Autodesk Fusion 360 part; units mm, degrees
(part 3 of 3)
  line L801 (-42.271, 19.322) -> (-42.57, 20.092)
  line L802 (-42.57, 20.092) -> (-42.917, 21.434)
  line L803 (-42.917, 21.434) -> (-43.042, 22.229)
  line L804 (-43.042, 22.229) -> (-43.116, 23.149)
  line L805 (-43.116, 23.149) -> (-43.116, 28.119)
  line L806 (-43.116, 28.119) -> (-42.942, 28.168)
  line L807 (-42.942, 28.168) -> (-42.843, 28.342)
  line L808 (-42.843, 28.342) -> (-42.843, 34.257)
  line L809 (-42.843, 34.257) -> (-42.967, 34.406)
  line L810 (-42.967, 34.406) -> (-43.887, 34.406)
  line L811 (-43.887, 34.406) -> (-44.011, 34.282)
  line L812 (-44.011, 34.282) -> (-44.011, 28.268)
  line L813 (-44.011, 28.268) -> (-43.936, 28.168)
  line L814 (-43.936, 28.168) -> (-43.837, 28.119)
  line L815 (-43.837, 28.119) -> (-43.837, 23.323)
  line L816 (-43.837, 23.323) -> (-43.762, 22.279)
  line L817 (-43.762, 22.279) -> (-43.564, 21.061)
  line L818 (-43.564, 21.061) -> (-43.315, 20.092)
  line L819 (-43.315, 20.092) -> (-42.942, 19.073)
  line L820 (-42.942, 19.073) -> (-42.57, 18.303)
  line L821 (-42.57, 18.303) -> (-42.172, 17.632)
  line L822 (-42.172, 17.632) -> (-41.799, 17.11)
  line L823 (-41.799, 17.11) -> (-41.153, 16.389)
  line L824 (-41.153, 16.389) -> (-40.383, 15.743)
  line L825 (-40.383, 15.743) -> (-39.712, 15.321)
  line L826 (-39.712, 15.321) -> (-39.687, 15.246)
  line L827 (-39.687, 15.246) -> (-39.761, 15.196)
  line L828 (-39.761, 15.196) -> (-40.532, 15.221)
  line L829 (-40.532, 15.221) -> (-41.079, 15.296)
  line L830 (-41.079, 15.296) -> (-41.6, 15.42)
  line L831 (-41.6, 15.42) -> (-42.545, 15.793)
  line L832 (-42.545, 15.793) -> (-43.191, 16.166)
  line L833 (-43.191, 16.166) -> (-43.837, 16.663)
  line L834 (-43.837, 16.663) -> (-44.409, 17.234)
  line L835 (-44.409, 17.234) -> (-44.756, 17.657)
  line L836 (-44.756, 17.657) -> (-45.353, 18.576)
  line L837 (-45.353, 18.576) -> (-45.8, 19.496)
  line L838 (-45.8, 19.496) -> (-46.123, 20.365)
  line L839 (-46.123, 20.365) -> (-46.347, 21.161)
  line L840 (-46.347, 21.161) -> (-46.496, 21.906)
  line L841 (-46.496, 21.906) -> (-46.62, 22.95)
  line L842 (-46.62, 22.95) -> (-46.645, 26.205)
  line L843 (-46.645, 26.205) -> (-46.546, 26.28)
  line L844 (-46.546, 26.28) -> (-46.496, 26.379)
  line L845 (-46.496, 26.379) -> (-46.496, 31.747)
  line L846 (-46.496, 31.747) -> (-46.67, 31.871)
  line L847 (-46.67, 31.871) -> (-47.515, 31.846)
  line L848 (-47.515, 31.846) -> (-47.614, 31.722)
  line L849 (-47.614, 31.722) -> (-47.614, 26.379)
  line L850 (-47.614, 26.379) -> (-47.54, 26.255)
  line L851 (-47.54, 26.255) -> (-47.416, 26.23)
  line L852 (-47.416, 26.23) -> (-47.366, 26.18)
  line L853 (-47.366, 26.18) -> (-47.366, 23.621)
  line L854 (-47.366, 23.621) -> (-47.316, 22.826)
  line L855 (-47.316, 22.826) -> (-47.117, 21.384)
  line L856 (-47.117, 21.384) -> (-46.918, 20.539)
  line L857 (-46.918, 20.539) -> (-46.67, 19.744)
  line L858 (-46.67, 19.744) -> (-46.372, 18.999)
  line L859 (-46.372, 18.999) -> (-45.9, 18.079)
  line L860 (-45.9, 18.079) -> (-45.452, 17.383)
  line L861 (-45.452, 17.383) -> (-45.005, 16.812)
  line L862 (-45.005, 16.812) -> (-44.483, 16.265)
  line L863 (-44.483, 16.265) -> (-43.862, 15.743)
  line L864 (-43.862, 15.743) -> (-42.843, 15.122)
  line L865 (-42.843, 15.122) -> (-41.725, 14.699)
  line L866 (-41.725, 14.699) -> (-41.054, 14.55)
  line L867 (-41.054, 14.55) -> (-40.507, 14.476)
  line L868 (-40.507, 14.476) -> (-39.563, 14.426)
  line L869 (-39.563, 14.426) -> (-38.792, 14.327)
  line L870 (-38.792, 14.327) -> (-34.816, 12.463)
  line L871 (-34.816, 12.463) -> (-34.766, 12.363)
  line L872 (-34.766, 12.363) -> (-35.313, 11.618)
  line L873 (-35.313, 11.618) -> (-35.437, 11.593)
  line L874 (-35.437, 11.593) -> (-38.917, 13.009)
  line L875 (-38.917, 13.009) -> (-42.371, 14.476)
  line L876 (-42.371, 14.476) -> (-42.445, 14.476)
  line L877 (-42.445, 14.476) -> (-42.4478, 14.4694)
  line L878 (-40.9545, 12.972) -> (-39.19, 12.239)
  line L879 (-39.19, 12.239) -> (-37.351, 11.518)
  line L880 (-37.351, 11.518) -> (-36.332, 11.071)
  line L881 (-36.332, 11.071) -> (-35.288, 10.673)
  line L882 (-35.288, 10.673) -> (-32.58, 9.53)
  line L883 (-32.58, 9.53) -> (-32.505, 9.53)
  line L884 (-32.505, 9.53) -> (-31.958, 9.282)
  line L885 (-31.958, 9.282) -> (-31.585, 9.158)
  line L886 (-31.585, 9.158) -> (-28.38, 7.791)
  line L887 (-28.38, 7.791) -> (-27.883, 7.542)
  line L888 (-27.883, 7.542) -> (-27.908, 7.468)
  line L889 (-27.908, 7.468) -> (-31.262, 5.852)
  line L890 (-31.262, 5.852) -> (-31.312, 5.803)
  line L891 (-31.312, 5.803) -> (-31.312, 5.728)
  line L892 (-31.312, 5.728) -> (-30.989, 5.057)
  line L893 (-30.989, 5.057) -> (-30.915, 5.057)
  line L894 (-30.915, 5.057) -> (-27.038, 7.02)
  line L895 (-27.038, 7.02) -> (-26.789, 7.07)
  line L896 (-26.789, 7.07) -> (-26.069, 6.722)
  line L897 (-26.069, 6.722) -> (-26.044, 6.623)
  line L898 (-26.044, 6.623) -> (-28.33, 5.455)
  line L899 (-28.33, 5.455) -> (-28.355, 5.331)
  line L900 (-28.355, 5.331) -> (-28.032, 4.684)
  line L901 (-28.032, 4.684) -> (-27.336, 5.007)
  line L902 (-27.336, 5.007) -> (-25.5, 5.9758)
  arc A12 (-8.7235, 42.6374) -> (-8.8988, 42.7975) centre (-25, 25) ccw
  arc A13 (-24.5, 1.0052) -> (-8.7441, 7.3437) centre (-25, 25) ccw
  arc A14 (-41.6193, 7.6853) -> (-25.5, 1.0052) centre (-25, 25) ccw
  arc A15 (-13.4958, 46.0631) -> (-13.8205, 46.2372) centre (-25, 25) ccw
  arc A16 (-14.7269, 46.6902) -> (-39.0593, 44.4509) centre (-25, 25) ccw
  arc A17 (-41.6193, 7.6853) -> (-25.5, 1.0052) centre (-25, 25) ccw
  arc A18 (-8.7235, 42.6374) -> (-8.8988, 42.7975) centre (-25, 25) ccw
  arc A19 (-24.5, 1.0052) -> (-8.7441, 7.3437) centre (-25, 25) ccw
  arc A20 (-41.6193, 7.6853) -> (-25.5, 1.0052) centre (-25, 25) ccw
  arc A21 (-13.4958, 46.0631) -> (-13.8205, 46.2372) centre (-25, 25) ccw
  arc A22 (-14.7269, 46.6902) -> (-39.0593, 44.4509) centre (-25, 25) ccw
  line L903 (-7.3062, 13.7316) -> (-2.9434, 15.5393)
  arc A23 (-8.7235, 42.6374) -> (-8.8988, 42.7975) centre (-25, 25) ccw
  line L904 (-46.9999, 15.4081) -> (-40.9545, 12.972)
  line L905 (-42.4478, 14.4694) -> (-47.4367, 16.4797)
  arc A24 (-40.0281, 43.7125) -> (-47.4367, 16.4797) centre (-25, 25) ccw
  arc A25 (-40.0281, 43.7125) -> (-47.4367, 16.4797) centre (-25, 25) ccw
  arc A26 (-6.803, 9.3517) -> (-2.9434, 15.5393) centre (-25, 25) ccw
  arc A27 (-2.5162, 16.6048) -> (-8.2028, 42.1422) centre (-25, 25) ccw
  arc A28 (-7.6077, 8.4619) -> (-6.9294, 9.2059) centre (-25, 25) ccw
  arc A29 (-46.9999, 15.4081) -> (-42.3147, 8.3807) centre (-25, 25) ccw
  arc A30 (-40.0281, 43.7125) -> (-47.4367, 16.4797) centre (-25, 25) ccw
  arc A31 (-40.0281, 43.7125) -> (-47.4367, 16.4797) centre (-25, 25) ccw
  arc A32 (-6.803, 9.3517) -> (-2.9434, 15.5393) centre (-25, 25) ccw
  arc A33 (-2.5162, 16.6048) -> (-8.2028, 42.1422) centre (-25, 25) ccw
  arc A34 (-7.6077, 8.4619) -> (-6.9294, 9.2059) centre (-25, 25) ccw
  arc A35 (-46.9999, 15.4081) -> (-42.3147, 8.3807) centre (-25, 25) ccw
  dimension "d11" = 51
  constraint concentric A3 A4
  measures "d11" diameter of A4
extrude "Extrude4" add sketch "Sketch4" along normal blind 3 contours A1 A2 A3
ref_plane "WorkPlane2" through (25, -25, 7.5) normal (0, 1, 0) x (-1, 0, 0)
sketch "Sketch6" plane through (0, -25, 0) normal (0, 1, 0) x (-1, 0, 0)
  line L0 (2.5, 6) -> (-52.5, 6)
  line L1 (-50.5, 6) -> (0.5, 6)
  line L2 (2.5, 6) -> (6.7012, 12)
  line L3 (4.7012, 12) -> (0.5, 6)
  line L4 (2.5, 6) -> (-52.5, 6)
  line L5 (2.5, 0) -> (-52.5, 0)
  line L6 (2.5, 4) -> (2.5, 0) construction
  line L7 (0.5, 6) -> (2.5, 6) construction
  line L8 (6.7012, 12) -> (4.7012, 12)
  dimension "d21" = 145
  dimension "d23" = 6
  constraint coincident L0.start L2.start
  constraint coincident L1.end L3.end
  constraint parallel L2 L3
  constraint coincident L5.start L6.end
  constraint horizontal L8
  measures "d21" angle of L2 L6
  measures "d23" distance of L0.start L8
revolve "Revolve1" add sketch "Sketch6" angle 15 about axis through (25, -25, -2.5) along (0, 0, -1)
pattern_circular "C-Pattern1" count 16 over 360 about axis through (25, -25, -2.5) along (0, 0, 1) of "Revolve1"
